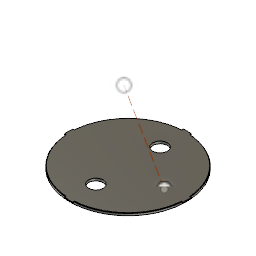
al-base-plate-deckel (Autodesk Fusion 360 design; units mm, degrees)
Autodesk Fusion 360 part; units mm, degrees
note: some values were not read from the file. Chosen so that the rebuilt part matches the saved one: which bodies a step acts on.
sketch "Skizze1" plane through (0, 0, 0) normal (0, 0, 1) x (1, 0, 0)
  circle A0 centre (0, 0) radius 80
extrude "Extrusion1" add sketch "Skizze1" along normal blind 10 makes body 1
fillet "Abrundung1" radius 2 1 edges at (-74.5862, -28.9292, 10) on bodies 1
sketch "Skizze2" plane through (0, 0, 0) normal (0, 1, 0) x (1, 0, 0)
  line L0 (45, 0) -> (-5, -86.6025) construction
ref_plane "Arbeitsebene1" through (-5, 0, 86.6025) normal (-0.5, 0, 0.866025) x (0, -1, 0)
sketch "Skizze3" plane through (-5, 0, 86.6025) normal (-0.5, 0, 0.866025) x (0, -1, 0)
  circle A0 centre (0, 0) radius 23
  circle A1 centre (0, 0) radius 20
extrude "Extrusion5" add sketch "Skizze3" against normal blind 110 separate body contours A0 | A1 makes body 2
combine "Kombinieren1" operation add target body 1 tool bodies 2
extrude "Extrusion6" cut sketch "Skizze3" against normal blind 50 bodies 1
fillet "Abrundung2" radius 4 3 edges at (65.7846, 0, 10) (-74.5862, -28.9292, 8) (-72.7215, 28.206, 10) on bodies 1
sketch "Skizze4" plane through (-5, 0, 86.6025) normal (-0.5, 0, 0.866025) x (0, -1, 0)
  circle A0 centre (0, 0) radius 15.75
extrude "Extrusion7" cut sketch "Skizze4" against normal blind 110 bodies 1
sketch "Skizze5" plane through (0, 0, 0) normal (0, 0, 1) x (1, 0, 0)
  circle A0 centre (0, 0) radius 160
extrude "Extrusion8" cut sketch "Skizze5" against normal blind 110 bodies 1
sketch "Skizze6" plane through (0, 0, 0) normal (0, 0, 1) x (1, 0, 0)
  line L0 (45, 0) -> (85, 0)
ref_plane "Arbeitsebene2" through (45, 0, 0) normal (1, 0, 0) x (0, 1, 0)
sketch "Skizze7" plane through (45, 0, 0) normal (1, 0, 0) x (0, 1, 0)
  line L0 (-4, 0) -> (-4, 1.7)
  line L1 (-4, 1.7) -> (-3.2, 3.3)
  line L2 (-3.2, 3.3) -> (-1, 5.5)
  line L3 (-1, 5.5) -> (1, 5.5)
  line L4 (1, 5.5) -> (3.2, 3.3)
  line L5 (3.2, 3.3) -> (4, 1.7)
  line L6 (4, 1.7) -> (4, 0)
  line L7 (4, 0) -> (-4, 0)
sweep "Sweeping1" cut profiles "Skizze7" path "Skizze6" along L0 section 1 bodies 1
sketch "Skizze8" plane through (0, 0, 0) normal (0, 0, 1) x (1, 0, 0)
  circle A0 centre (0, 0) radius 72.5
extrude "Extrusion9" cut sketch "Skizze8" along normal blind 3 bodies 1
sketch "Skizze9" plane through (0, 0, 0) normal (0, 0, 1) x (1, 0, 0)
  line L0 (72.2241, -6.3188) -> (73.7184, -6.4495)
  arc A0 (73.7184, -6.4495) -> (73.7184, 6.4495) centre (0, 0) ccw
  line L1 (73.7184, 6.4495) -> (72.2241, 6.3188)
  arc A1 (72.2241, -6.3188) -> (72.2241, 6.3188) centre (0, 0) ccw
  line L2 (6.3188, 72.2241) -> (6.4495, 73.7184)
  arc A2 (6.4495, 73.7184) -> (-6.4495, 73.7184) centre (0, 0) ccw
  line L3 (-6.4495, 73.7184) -> (-6.3188, 72.2241)
  arc A3 (6.3188, 72.2241) -> (-6.3188, 72.2241) centre (0, 0) ccw
  line L4 (-72.2241, 6.3188) -> (-73.7184, 6.4495)
  arc A4 (-73.7184, 6.4495) -> (-73.7184, -6.4495) centre (0, 0) ccw
  line L5 (-73.7184, -6.4495) -> (-72.2241, -6.3188)
  arc A5 (-72.2241, 6.3188) -> (-72.2241, -6.3188) centre (0, 0) ccw
  line L6 (-6.3188, -72.2241) -> (-6.4495, -73.7184)
  arc A6 (-6.4495, -73.7184) -> (6.4495, -73.7184) centre (0, 0) ccw
  line L7 (6.4495, -73.7184) -> (6.3188, -72.2241)
  arc A7 (-6.3188, -72.2241) -> (6.3188, -72.2241) centre (0, 0) ccw
extrude "Extrusion10" cut sketch "Skizze9" along normal blind 3 bodies 1
sketch "Skizze10" plane through (0, 0, 0) normal (0, 0, 1) x (1, 0, 0)
  line L0 (72.2241, -6.3188) -> (73.7184, -6.4495)
  arc A0 (73.7184, -6.4495) -> (69.5373, 25.3095) centre (0, 0) ccw
  line L1 (69.5373, 25.3095) -> (68.1277, 24.7965)
  arc A1 (72.2241, -6.3188) -> (68.1277, 24.7965) centre (0, 0) ccw
  line L2 (6.3188, 72.2241) -> (6.4495, 73.7184)
  arc A2 (6.4495, 73.7184) -> (-25.3095, 69.5373) centre (0, 0) ccw
  line L3 (-25.3095, 69.5373) -> (-24.7965, 68.1277)
  arc A3 (6.3188, 72.2241) -> (-24.7965, 68.1277) centre (0, 0) ccw
  line L4 (-72.2241, 6.3188) -> (-73.7184, 6.4495)
  arc A4 (-73.7184, 6.4495) -> (-69.5373, -25.3095) centre (0, 0) ccw
  line L5 (-69.5373, -25.3095) -> (-68.1277, -24.7965)
  arc A5 (-72.2241, 6.3188) -> (-68.1277, -24.7965) centre (0, 0) ccw
  line L6 (-6.3188, -72.2241) -> (-6.4495, -73.7184)
  arc A6 (-6.4495, -73.7184) -> (25.3095, -69.5373) centre (0, 0) ccw
  line L7 (25.3095, -69.5373) -> (24.7965, -68.1277)
  arc A7 (-6.3188, -72.2241) -> (24.7965, -68.1277) centre (0, 0) ccw
extrude "Extrusion11" cut sketch "Skizze10" along normal blind 1.25 from surface at 1.75 bodies 1
sketch "Skizze11" plane through (0, 0, 0) normal (0, 0, 1) x (1, 0, 0)
  circle A0 centre (0, 0) radius 72.2
extrude "Extrusion12" add sketch "Skizze11" along normal blind 3 separate body makes body 3
fillet "Abrundung3" radius 0.5 1 edges at (-67.314, -26.1086, 3) on bodies 3
sketch "Skizze12" plane through (0, 0, 0) normal (0, 0, 1) x (1, 0, 0)
  line L0 (71.0266, -4.9667) -> (73.5205, -5.1411)
  arc A0 (73.5205, -5.1411) -> (73.5205, 5.1411) centre (0, 0) ccw
  line L1 (73.5205, 5.1411) -> (71.0266, 4.9667)
  arc A1 (71.0266, -4.9667) -> (71.0266, 4.9667) centre (0, 0) ccw
  line L2 (4.9667, 71.0266) -> (5.1411, 73.5205)
  arc A2 (5.1411, 73.5205) -> (-5.1411, 73.5205) centre (0, 0) ccw
  line L3 (-5.1411, 73.5205) -> (-4.9667, 71.0266)
  arc A3 (4.9667, 71.0266) -> (-4.9667, 71.0266) centre (0, 0) ccw
  line L4 (-71.0266, 4.9667) -> (-73.5205, 5.1411)
  arc A4 (-73.5205, 5.1411) -> (-73.5205, -5.1411) centre (0, 0) ccw
  line L5 (-73.5205, -5.1411) -> (-71.0266, -4.9667)
  arc A5 (-71.0266, 4.9667) -> (-71.0266, -4.9667) centre (0, 0) ccw
  line L6 (-4.9667, -71.0266) -> (-5.1411, -73.5205)
  arc A6 (-5.1411, -73.5205) -> (5.1411, -73.5205) centre (0, 0) ccw
  line L7 (5.1411, -73.5205) -> (4.9667, -71.0266)
  arc A7 (-4.9667, -71.0266) -> (4.9667, -71.0266) centre (0, 0) ccw
extrude "Extrusion13" add sketch "Skizze12" along normal blind 1.1 from surface at 1.9 separate body makes body 4 at (-72.7424, 3.9409, 1.9) makes body 5 at (-3.9409, 72.7424, 1.9) makes body 6 at (72.7424, 3.9409, 1.9) makes body 7 at (0.5522, -72.8469, 1.9)
combine "Kombinieren2" operation add target body 3 tool bodies 4 5 6 7
sketch "Skizze13" plane through (0, 0, 0) normal (0, 0, 1) x (1, 0, 0)
  circle A0 centre (0, 39.875) radius 9
  circle A1 centre (0, -39.875) radius 9
extrude "Extrusion14" cut sketch "Skizze13" along normal blind 3 bodies 3
delete_body "Körper entfernen1" bodies 1
equation "base_plate_diameter = 160 mm" comment "Durchmesser der runden Basis-Platte"
equation "base_plate_height = 10 mm" comment "Höhe der runden Basis-Platte"
equation "base_plate_rounding = 2 mm" comment "Abrundung der oberen Basis-Platte-Kante (Kreis)"
equation "leg_outer_diameter = 46 mm" comment "Aussendurchmesser der Röhre"
equation "ring_inner_diameter = 40 mm" comment "Aussendurchmesser des oberen Röhrensegments (Stufenabsatz)"
equation "ring_extrude_depth = 50 mm" comment "Länge des oberen (dünnen) Röhrensegments / Stufenabsatz"
equation "hole_inner_diameter = 31.5 mm" comment "Innendurchmesser der Röhre (Loch)"
equation "leg_length = 100 mm" comment "Laenge der Röhre"
equation "leg_angle = 120 deg" comment "Winkel des Beines zur XY-Ebene (Innenwinkel an der Platte)"
equation "leg_offset = 45 mm" comment "Abstand des Bein-Fußpunktes vom Plattenmittelpunkt"
equation "leg_plate_rounding = 4 mm" comment "Abrundung der Kante: Bein und Platte (wird bei Solver-Problemen automatisch verkleinert)"
equation "cable_channel_width = 8 mm" comment "Breite des unterseitigen Kabelkanals"
equation "cable_channel_depth = 5.5 mm" comment "Gesamttiefe des unterseitigen Kabelkanals"
equation "cable_channel_vertical_height = 2.5 mm" comment "Höhe des senkrechten Wand-Abschnitts des Kabelkanals"
equation "cable_channel_edge_chamfer = 0.8 mm" comment "Abfasung der Kante zwischen senkrechter Wand und 45°-Dach im Kabelkanal"
equation "cover_plate_diameter = 145 mm" comment "Durchmesser der unterseitigen Abdeckplatte (Vertiefung)"
equation "cover_plate_thickness = 3 mm" comment "Dicke der unterseitigen Abdeckplatte"
equation "finger_grip_diameter = 18 mm" comment "Durchmesser der Finger-Vertiefungen zum Drehen der Abdeckplatte"
equation "finger_grip_depth = 1.5 mm" comment "Tiefe der Finger-Vertiefungen an der Unterseite der Abdeckplatte"
equation "clamp_recess_width = 22 mm" comment "Breite der Klemmsteg-Vertiefung quer zum Kanal"
equation "clamp_recess_length = 12 mm" comment "Länge der Klemmsteg-Vertiefung entlang des Kanals"
equation "clamp_recess_depth = 2.5 mm" comment "Tiefe der Klemmsteg-Vertiefung an der Unterseite"
equation "strain_relief_screw_diameter = 2.6 mm" comment "Bohrungsdurchmesser für M3-Zugsicherungsschellen"
equation "strain_relief_screw_depth = 6 mm" comment "Bohrungstiefe für M3-Zugsicherungsschellen"
equation "d25 = base_plate_height"
equation "d28 = base_plate_rounding"
equation "d36 = -( leg_length + base_plate_height )"
equation "d38 = -ring_extrude_depth"
equation "d41 = leg_plate_rounding"
equation "d42 = -leg_length - base_plate_height"
equation "d44 = -( leg_length + base_plate_height )"
equation "d53 = cover_plate_thickness"
equation "d55 = cover_plate_thickness"
equation "d60 = cover_plate_thickness"
equation "d67 = cover_plate_thickness"
